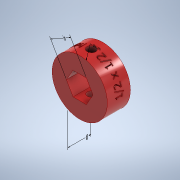
# Autodesk Inventor part: 1_2x1_2x1-1_2HexBearing
Saved by Autodesk Inventor 2022.2 (Build 262287000, 287)
## iProperties
Created: 2020-11-08
Part Number: 1_2x1_2x1-1_2HexBearing
Material: PC/ABS Plastic
Document SubType Name: Modeling
Designer: robst
Density: 0.357273 g/cm^3
Appearance: Red
Author: robst
Autodesk Inventor part; units mm, degrees
ref_plane "YZ Plane" through (0, 0, 0) normal (1, 0, 0) x (0, 1, 0)
ref_plane "XZ Plane" through (0, 0, 0) normal (0, 1, 0) x (-1, 0, 0)
ref_plane "XY Plane" through (0, 0, 0) normal (0, 0, 1) x (1, 0, 0)
sketch "Sketch1" plane through (0, 0, 0) normal (0, 0, 1) x (1, 0, 0)
  line L0 (3.6662, 6.35) -> (7.3323, 0)
  line L1 (7.3323, 0) -> (3.6662, -6.35)
  line L2 (3.6662, -6.35) -> (-3.6662, -6.35)
  line L3 (-3.6662, -6.35) -> (-7.3323, 0)
  line L4 (-7.3323, 0) -> (-3.6662, 6.35)
  line L5 (-3.6662, 6.35) -> (3.6662, 6.35)
  circle A0 centre (0, 0) radius 15.2146
  circle A1 centre (0, 0) radius 7.3323 construction
  dimension "d0" = 12.7
  dimension "d2" = 30.4292
  dimension "d3" = 7.8822
  constraints: 12 end point, 3 coincident, 1 centre point, 1 horizontal, 1 horizontal alignment, 15 other
  measures "d0" distance between parallel lines of L2 L5
  measures "d2" diameter of A0
extrude "Extrusion1" add sketch "Sketch1" against normal blind 12.7
ref_plane "Work Plane1" through (0, 15.2146, 0) normal (0, 1, 0) x (-1, 0, 0)
sketch "Sketch2" plane through (0, 15.2146, 0) normal (0, 1, 0) x (-1, 0, 0)
  line L0 (0, -6.35) -> (-25.4, -6.35) construction
  line L1 (15.2146, 0) -> (-15.2146, 0) construction
  line L2 (-22.9639, -8.255) -> (-24.8226, -8.255)
  line L3 (-24.8226, -8.255) -> (-24.8226, -7.866)
  line L4 (-24.8226, -7.866) -> (-24.131, -7.866)
  line L5 (-24.131, -7.866) -> (-24.131, -5.3126)
  line L6 (-24.131, -5.3126) -> (-24.8226, -5.3126)
  line L7 (-24.8226, -5.3126) -> (-24.8226, -4.9637)
  spline S0 degree 2 poles (-24.8226, -4.9637) (-24.4305, -4.9637) (-24.06, -4.7414) (-24.0353, -4.4326) knots 0 0 0 1 2 2 2
  line L8 (-24.0353, -4.4326) -> (-23.6401, -4.4326)
  line L9 (-23.6401, -4.4326) -> (-23.6401, -7.866)
  line L10 (-23.6401, -7.866) -> (-22.9639, -7.866)
  line L11 (-22.9639, -7.866) -> (-22.9639, -8.255)
  line L12 (-20.6792, -4.2752) -> (-22.1705, -9.0825)
  line L13 (-22.1705, -9.0825) -> (-22.6027, -9.0825)
  line L14 (-22.6027, -9.0825) -> (-21.1176, -4.2752)
  line L15 (-21.1176, -4.2752) -> (-20.6792, -4.2752)
  line L16 (-17.9097, -8.255) -> (-20.2593, -8.255)
  line L17 (-20.2593, -8.255) -> (-20.2593, -7.7147)
  spline S1 degree 2 poles (-20.2593, -7.7147) (-20.0061, -7.4769) (-19.5553, -7.0354) (-19.3392, -6.7977) knots 0 0 0 1 2 2 2
  spline S2 degree 2 poles (-19.3392, -6.7977) (-18.9039, -6.3191) (-18.5858, -5.7448) (-18.5858, -5.4392) knots 0 0 0 1 2 2 2
  spline S3 degree 2 poles (-18.5858, -5.4392) (-18.5858, -5.2786) (-18.6846, -5.0378) (-18.7742, -4.9606) knots 0 0 0 1 2 2 2
  spline S4 degree 2 poles (-18.7742, -4.9606) (-18.8637, -4.8834) (-19.0984, -4.8062) (-19.2404, -4.8062) knots 0 0 0 1 2 2 2
  spline S5 degree 2 poles (-19.2404, -4.8062) (-19.3762, -4.8062) (-19.6541, -4.8742) (-19.7807, -4.9267) knots 0 0 0 1 2 2 2
  spline S6 degree 2 poles (-19.7807, -4.9267) (-19.8888, -4.9699) (-20.0895, -5.0934) (-20.1512, -5.1366) knots 0 0 0 1 2 2 2
  line L18 (-20.1512, -5.1366) -> (-20.179, -5.1366)
  line L19 (-20.179, -5.1366) -> (-20.179, -4.5932)
  spline S7 degree 2 poles (-20.179, -4.5932) (-20.0215, -4.516) (-19.4565, -4.3647) (-19.2033, -4.3647) knots 0 0 0 1 2 2 2
  spline S8 degree 2 poles (-19.2033, -4.3647) (-18.6692, -4.3647) (-18.0671, -4.9297) (-18.0671, -5.4114) knots 0 0 0 1 2 2 2
  spline S9 degree 2 poles (-18.0671, -5.4114) (-18.0671, -5.6368) (-18.1721, -6.0135) (-18.2647, -6.174) knots 0 0 0 1 2 2 2
  spline S10 degree 2 poles (-18.2647, -6.174) (-18.3574, -6.3407) (-18.626, -6.668) (-18.7742, -6.8255) knots 0 0 0 1 2 2 2
  spline S11 degree 2 poles (-18.7742, -6.8255) (-19.015, -7.0879) (-19.6047, -7.6498) (-19.7807, -7.8135) knots 0 0 0 1 2 2 2
  line L20 (-19.7807, -7.8135) -> (-17.9097, -7.8135)
  line L21 (-17.9097, -7.8135) -> (-17.9097, -8.255)
  line L22 (-13.4729, -8.255) -> (-14.0626, -8.255)
  line L23 (-14.0626, -8.255) -> (-14.7573, -7.1805)
  line L24 (-14.7573, -7.1805) -> (-15.4705, -8.255)
  line L25 (-15.4705, -8.255) -> (-16.017, -8.255)
  line L26 (-16.017, -8.255) -> (-15.0259, -6.8378)
  line L27 (-15.0259, -6.8378) -> (-16.0078, -5.396)
  line L28 (-16.0078, -5.396) -> (-15.418, -5.396)
  line L29 (-15.418, -5.396) -> (-14.7264, -6.4612)
  line L30 (-14.7264, -6.4612) -> (-14.0194, -5.396)
  line L31 (-14.0194, -5.396) -> (-13.4729, -5.396)
  line L32 (-13.4729, -5.396) -> (-14.4578, -6.807)
  line L33 (-14.4578, -6.807) -> (-13.4729, -8.255)
  line L34 (-9.3758, -8.255) -> (-11.2345, -8.255)
  line L35 (-11.2345, -8.255) -> (-11.2345, -7.866)
  line L36 (-11.2345, -7.866) -> (-10.5429, -7.866)
  line L37 (-10.5429, -7.866) -> (-10.5429, -5.3126)
  line L38 (-10.5429, -5.3126) -> (-11.2345, -5.3126)
  line L39 (-11.2345, -5.3126) -> (-11.2345, -4.9637)
  spline S12 degree 2 poles (-11.2345, -4.9637) (-10.8423, -4.9637) (-10.4718, -4.7414) (-10.4471, -4.4326) knots 0 0 0 1 2 2 2
  line L40 (-10.4471, -4.4326) -> (-10.0519, -4.4326)
  line L41 (-10.0519, -4.4326) -> (-10.0519, -7.866)
  line L42 (-10.0519, -7.866) -> (-9.3758, -7.866)
  line L43 (-9.3758, -7.866) -> (-9.3758, -8.255)
  line L44 (-7.091, -4.2752) -> (-8.5823, -9.0825)
  line L45 (-8.5823, -9.0825) -> (-9.0145, -9.0825)
  line L46 (-9.0145, -9.0825) -> (-7.5294, -4.2752)
  line L47 (-7.5294, -4.2752) -> (-7.091, -4.2752)
  line L48 (-4.3215, -8.255) -> (-6.6711, -8.255)
  line L49 (-6.6711, -8.255) -> (-6.6711, -7.7147)
  spline S13 degree 2 poles (-6.6711, -7.7147) (-6.4179, -7.4769) (-5.9671, -7.0354) (-5.751, -6.7977) knots 0 0 0 1 2 2 2
  spline S14 degree 2 poles (-5.751, -6.7977) (-5.3157, -6.3191) (-4.9977, -5.7448) (-4.9977, -5.4392) knots 0 0 0 1 2 2 2
  spline S15 degree 2 poles (-4.9977, -5.4392) (-4.9977, -5.2786) (-5.0965, -5.0378) (-5.186, -4.9606) knots 0 0 0 1 2 2 2
  spline S16 degree 2 poles (-5.186, -4.9606) (-5.2755, -4.8834) (-5.5102, -4.8062) (-5.6522, -4.8062) knots 0 0 0 1 2 2 2
  spline S17 degree 2 poles (-5.6522, -4.8062) (-5.7881, -4.8062) (-6.0659, -4.8742) (-6.1925, -4.9267) knots 0 0 0 1 2 2 2
  spline S18 degree 2 poles (-6.1925, -4.9267) (-6.3006, -4.9699) (-6.5013, -5.0934) (-6.563, -5.1366) knots 0 0 0 1 2 2 2
  line L50 (-6.563, -5.1366) -> (-6.5908, -5.1366)
  line L51 (-6.5908, -5.1366) -> (-6.5908, -4.5932)
  spline S19 degree 2 poles (-6.5908, -4.5932) (-6.4334, -4.516) (-5.8683, -4.3647) (-5.6152, -4.3647) knots 0 0 0 1 2 2 2
  spline S20 degree 2 poles (-5.6152, -4.3647) (-5.081, -4.3647) (-4.479, -4.9297) (-4.479, -5.4114) knots 0 0 0 1 2 2 2
  spline S21 degree 2 poles (-4.479, -5.4114) (-4.479, -5.6368) (-4.5839, -6.0135) (-4.6766, -6.174) knots 0 0 0 1 2 2 2
  spline S22 degree 2 poles (-4.6766, -6.174) (-4.7692, -6.3407) (-5.0378, -6.668) (-5.186, -6.8255) knots 0 0 0 1 2 2 2
  spline S23 degree 2 poles (-5.186, -6.8255) (-5.4268, -7.0879) (-6.0165, -7.6498) (-6.1925, -7.8135) knots 0 0 0 1 2 2 2
  line L52 (-6.1925, -7.8135) -> (-4.3215, -7.8135)
  line L53 (-4.3215, -7.8135) -> (-4.3215, -8.255)
  line L54 (6.6855, -8.255) -> (6.2039, -8.255)
  line L55 (6.2039, -8.255) -> (6.2039, -6.6248)
  spline S24 degree 2 poles (6.2039, -6.6248) (6.2039, -6.4272) (6.1668, -6.0876) (6.1112, -5.9857) knots 0 0 0 1 2 2 2
  spline S25 degree 2 poles (6.1112, -5.9857) (6.0526, -5.8776) (5.8426, -5.7726) (5.6635, -5.7726) knots 0 0 0 1 2 2 2
  spline S26 degree 2 poles (5.6635, -5.7726) (5.4845, -5.7726) (5.1047, -5.9641) (4.9225, -6.1184) knots 0 0 0 1 2 2 2
  line L56 (4.9225, -6.1184) -> (4.9225, -8.255)
  line L57 (4.9225, -8.255) -> (4.4409, -8.255)
  line L58 (4.4409, -8.255) -> (4.4409, -4.2752)
  line L59 (4.4409, -4.2752) -> (4.9225, -4.2752)
  line L60 (4.9225, -4.2752) -> (4.9225, -5.714)
  spline S27 degree 2 poles (4.9225, -5.714) (5.1387, -5.5195) (5.5555, -5.3157) (5.7901, -5.3157) knots 0 0 0 1 2 2 2
  spline S28 degree 2 poles (5.7901, -5.3157) (6.21, -5.3157) (6.6855, -5.8714) (6.6855, -6.3994) knots 0 0 0 1 2 2 2
  line L61 (6.6855, -6.3994) -> (6.6855, -8.255)
  spline S29 degree 2 poles (8.6029, -8.3198) (7.9174, -8.3198) (7.1641, -7.551) (7.1641, -6.8409) knots 0 0 0 1 2 2 2
  spline S30 degree 2 poles (7.1641, -6.8409) (7.1641, -6.1431) (7.8958, -5.3157) (8.4855, -5.3157) knots 0 0 0 1 2 2 2
  spline S31 degree 2 poles (8.4855, -5.3157) (8.7511, -5.3157) (9.1617, -5.4701) (9.313, -5.6337) knots 0 0 0 1 2 2 2
  spline S32 degree 2 poles (9.313, -5.6337) (9.4674, -5.7973) (9.631, -6.2697) (9.631, -6.6124) knots 0 0 0 1 2 2 2
  line L62 (9.631, -6.6124) -> (9.631, -6.8749)
  line L63 (9.631, -6.8749) -> (7.6519, -6.8749)
  spline S33 degree 2 poles (7.6519, -6.8749) (7.6519, -7.372) (8.1521, -7.8999) (8.5967, -7.8999) knots 0 0 0 1 2 2 2
  spline S34 degree 2 poles (8.5967, -7.8999) (8.7541, -7.8999) (9.0598, -7.8289) (9.1833, -7.7733) knots 0 0 0 1 2 2 2
  spline S35 degree 2 poles (9.1833, -7.7733) (9.313, -7.7116) (9.4921, -7.6035) (9.5507, -7.5541) knots 0 0 0 1 2 2 2
  line L64 (9.5507, -7.5541) -> (9.5785, -7.5541)
  line L65 (9.5785, -7.5541) -> (9.5785, -8.079)
  spline S36 degree 2 poles (9.5785, -8.079) (9.4952, -8.113) (9.242, -8.2118) (9.1432, -8.2396) knots 0 0 0 1 2 2 2
  spline S37 degree 2 poles (9.1432, -8.2396) (9.0042, -8.2797) (8.7758, -8.3198) (8.6029, -8.3198) knots 0 0 0 1 2 2 2
  spline S38 degree 2 poles (9.1617, -6.5075) (9.1555, -6.3129) (9.0753, -6.0289) (8.9981, -5.9332) knots 0 0 0 1 2 2 2
  spline S39 degree 2 poles (8.9981, -5.9332) (8.9147, -5.8251) (8.6523, -5.7109) (8.4577, -5.7109) knots 0 0 0 1 2 2 2
  spline S40 degree 2 poles (8.4577, -5.7109) (8.2663, -5.7109) (7.9977, -5.8251) (7.8866, -5.9363) knots 0 0 0 1 2 2 2
  spline S41 degree 2 poles (7.8866, -5.9363) (7.7785, -6.0505) (7.6673, -6.3253) (7.6519, -6.5075) knots 0 0 0 1 2 2 2
  line L66 (7.6519, -6.5075) -> (9.1617, -6.5075)
  line L67 (12.3388, -8.255) -> (11.749, -8.255)
  line L68 (11.749, -8.255) -> (11.0544, -7.1805)
  line L69 (11.0544, -7.1805) -> (10.3411, -8.255)
  line L70 (10.3411, -8.255) -> (9.7946, -8.255)
  line L71 (9.7946, -8.255) -> (10.7857, -6.8378)
  line L72 (10.7857, -6.8378) -> (9.8039, -5.396)
  line L73 (9.8039, -5.396) -> (10.3936, -5.396)
  line L74 (10.3936, -5.396) -> (11.0852, -6.4612)
  line L75 (11.0852, -6.4612) -> (11.7923, -5.396)
  line L76 (11.7923, -5.396) -> (12.3388, -5.396)
  line L77 (12.3388, -5.396) -> (11.3538, -6.807)
  line L78 (11.3538, -6.807) -> (12.3388, -8.255)
  spline S42 degree 2 poles (16.7447, -6.7792) (16.7447, -7.48) (16.0654, -8.3353) (15.5529, -8.3353) knots 0 0 0 1 2 2 2
  spline S43 degree 2 poles (15.5529, -8.3353) (15.3213, -8.3353) (14.9909, -8.221) (14.8304, -8.1222) knots 0 0 0 1 2 2 2
  line L79 (14.8304, -8.1222) -> (14.7995, -8.255)
  line L80 (14.7995, -8.255) -> (14.3487, -8.255)
  line L81 (14.3487, -8.255) -> (14.3487, -4.2752)
  line L82 (14.3487, -4.2752) -> (14.8304, -4.2752)
  line L83 (14.8304, -4.2752) -> (14.8304, -5.6954)
  spline S44 degree 2 poles (14.8304, -5.6954) (15.0126, -5.5318) (15.4355, -5.3157) (15.7042, -5.3157) knots 0 0 0 1 2 2 2
  spline S45 degree 2 poles (15.7042, -5.3157) (16.1889, -5.3157) (16.7447, -6.0906) (16.7447, -6.7792) knots 0 0 0 1 2 2 2
  spline S46 degree 2 poles (16.2476, -6.8162) (16.2476, -6.3037) (15.9357, -5.7726) (15.5899, -5.7726) knots 0 0 0 1 2 2 2
  spline S47 degree 2 poles (15.5899, -5.7726) (15.3954, -5.7726) (14.994, -5.9579) (14.8304, -6.0999) knots 0 0 0 1 2 2 2
  line L84 (14.8304, -6.0999) -> (14.8304, -7.7394)
  spline S48 degree 2 poles (14.8304, -7.7394) (15.0126, -7.8289) (15.2935, -7.903) (15.4602, -7.903) knots 0 0 0 1 2 2 2
  spline S49 degree 2 poles (15.4602, -7.903) (15.8277, -7.903) (16.2476, -7.3812) (16.2476, -6.8162) knots 0 0 0 1 2 2 2
  line L85 (19.4678, -8.255) -> (18.9862, -8.255)
  line L86 (18.9862, -8.255) -> (18.9862, -7.9401)
  spline S50 degree 2 poles (18.9862, -7.9401) (18.7639, -8.1346) (18.3656, -8.3353) (18.1186, -8.3353) knots 0 0 0 1 2 2 2
  spline S51 degree 2 poles (18.1186, -8.3353) (17.9333, -8.3353) (17.603, -8.2118) (17.4826, -8.079) knots 0 0 0 1 2 2 2
  spline S52 degree 2 poles (17.4826, -8.079) (17.3591, -7.9462) (17.2232, -7.5418) (17.2232, -7.2516) knots 0 0 0 1 2 2 2
  line L87 (17.2232, -7.2516) -> (17.2232, -5.396)
  line L88 (17.2232, -5.396) -> (17.7049, -5.396)
  line L89 (17.7049, -5.396) -> (17.7049, -7.0262)
  spline S53 degree 2 poles (17.7049, -7.0262) (17.7049, -7.2546) (17.7388, -7.5541) (17.7975, -7.6653) knots 0 0 0 1 2 2 2
  spline S54 degree 2 poles (17.7975, -7.6653) (17.8562, -7.7764) (18.0568, -7.8783) (18.2452, -7.8783) knots 0 0 0 1 2 2 2
  spline S55 degree 2 poles (18.2452, -7.8783) (18.4212, -7.8783) (18.8195, -7.6776) (18.9862, -7.5325) knots 0 0 0 1 2 2 2
  line L90 (18.9862, -7.5325) -> (18.9862, -5.396)
  line L91 (18.9862, -5.396) -> (19.4678, -5.396)
  line L92 (19.4678, -5.396) -> (19.4678, -8.255)
  spline S56 degree 2 poles (20.9375, -8.3229) (20.6504, -8.3229) (20.1533, -8.1685) (19.9896, -8.0821) knots 0 0 0 1 2 2 2
  line L93 (19.9896, -8.0821) -> (19.9896, -7.5418)
  line L94 (19.9896, -7.5418) -> (20.0143, -7.5418)
  spline S57 degree 2 poles (20.0143, -7.5418) (20.0761, -7.5912) (20.2428, -7.7085) (20.3818, -7.7733) knots 0 0 0 1 2 2 2
  spline S58 degree 2 poles (20.3818, -7.7733) (20.5022, -7.832) (20.7986, -7.9185) (20.956, -7.9185) knots 0 0 0 1 2 2 2
  spline S59 degree 2 poles (20.956, -7.9185) (21.0703, -7.9185) (21.3327, -7.866) (21.3945, -7.8227) knots 0 0 0 1 2 2 2
  spline S60 degree 2 poles (21.3945, -7.8227) (21.484, -7.7641) (21.5643, -7.6313) (21.5643, -7.4955) knots 0 0 0 1 2 2 2
  spline S61 degree 2 poles (21.5643, -7.4955) (21.5643, -7.3257) (21.379, -7.1497) (21.1413, -7.091) knots 0 0 0 1 2 2 2
  spline S62 degree 2 poles (21.1413, -7.091) (21.0487, -7.0694) (20.7523, -7.0076) (20.6257, -6.9737) knots 0 0 0 1 2 2 2
  spline S63 degree 2 poles (20.6257, -6.9737) (20.2984, -6.878) (20.002, -6.4828) (20.002, -6.2018) knots 0 0 0 1 2 2 2
  spline S64 degree 2 poles (20.002, -6.2018) (20.002, -5.8128) (20.5855, -5.328) (21.0672, -5.328) knots 0 0 0 1 2 2 2
  spline S65 degree 2 poles (21.0672, -5.328) (21.3049, -5.328) (21.7866, -5.4454) (21.9502, -5.5349) knots 0 0 0 1 2 2 2
  line L95 (21.9502, -5.5349) -> (21.9502, -6.0505)
  line L96 (21.9502, -6.0505) -> (21.9255, -6.0505)
  spline S66 degree 2 poles (21.9255, -6.0505) (21.7403, -5.9023) (21.2895, -5.7325) (21.0579, -5.7325) knots 0 0 0 1 2 2 2
  spline S67 degree 2 poles (21.0579, -5.7325) (20.8202, -5.7325) (20.4929, -5.9332) (20.4929, -6.1339) knots 0 0 0 1 2 2 2
  spline S68 degree 2 poles (20.4929, -6.1339) (20.4929, -6.316) (20.6874, -6.492) (20.9035, -6.5476) knots 0 0 0 1 2 2 2
  spline S69 degree 2 poles (20.9035, -6.5476) (21.0085, -6.5754) (21.274, -6.631) (21.4192, -6.6649) knots 0 0 0 1 2 2 2
  spline S70 degree 2 poles (21.4192, -6.6649) (21.7341, -6.7452) (22.0552, -7.1126) (22.0552, -7.4306) knots 0 0 0 1 2 2 2
  spline S71 degree 2 poles (22.0552, -7.4306) (22.0552, -7.6159) (21.9101, -7.9432) (21.768, -8.0636) knots 0 0 0 1 2 2 2
  spline S72 degree 2 poles (21.768, -8.0636) (21.6168, -8.1902) (21.2308, -8.3229) (20.9375, -8.3229) knots 0 0 0 1 2 2 2
  line L97 (24.7475, -8.255) -> (24.2659, -8.255)
  line L98 (24.2659, -8.255) -> (24.2659, -6.6248)
  spline S73 degree 2 poles (24.2659, -6.6248) (24.2659, -6.4272) (24.2288, -6.0876) (24.1732, -5.9857) knots 0 0 0 1 2 2 2
  spline S74 degree 2 poles (24.1732, -5.9857) (24.1146, -5.8776) (23.9046, -5.7726) (23.7255, -5.7726) knots 0 0 0 1 2 2 2
  spline S75 degree 2 poles (23.7255, -5.7726) (23.5465, -5.7726) (23.1667, -5.9641) (22.9845, -6.1184) knots 0 0 0 1 2 2 2
  line L99 (22.9845, -6.1184) -> (22.9845, -8.255)
  line L100 (22.9845, -8.255) -> (22.5029, -8.255)
  line L101 (22.5029, -8.255) -> (22.5029, -4.2752)
  line L102 (22.5029, -4.2752) -> (22.9845, -4.2752)
  line L103 (22.9845, -4.2752) -> (22.9845, -5.714)
  spline S76 degree 2 poles (22.9845, -5.714) (23.2007, -5.5195) (23.6175, -5.3157) (23.8521, -5.3157) knots 0 0 0 1 2 2 2
  spline S77 degree 2 poles (23.8521, -5.3157) (24.272, -5.3157) (24.7475, -5.8714) (24.7475, -6.3994) knots 0 0 0 1 2 2 2
  line L104 (24.7475, -6.3994) -> (24.7475, -8.255)
  line L105 (25.9146, -8.255) -> (25.4329, -8.255)
  line L106 (25.4329, -8.255) -> (25.4329, -5.396)
  line L107 (25.4329, -5.396) -> (25.9146, -5.396)
  line L108 (25.9146, -5.396) -> (25.9146, -8.255)
  line L109 (25.9486, -4.9205) -> (25.4021, -4.9205)
  line L110 (25.4021, -4.9205) -> (25.4021, -4.4203)
  line L111 (25.4021, -4.4203) -> (25.9486, -4.4203)
  line L112 (25.9486, -4.4203) -> (25.9486, -4.9205)
  line L113 (28.8663, -8.255) -> (28.3846, -8.255)
  line L114 (28.3846, -8.255) -> (28.3846, -6.6248)
  spline S78 degree 2 poles (28.3846, -6.6248) (28.3846, -6.4272) (28.3476, -6.0876) (28.292, -5.9857) knots 0 0 0 1 2 2 2
  spline S79 degree 2 poles (28.292, -5.9857) (28.2333, -5.8776) (28.0234, -5.7726) (27.8443, -5.7726) knots 0 0 0 1 2 2 2
  spline S80 degree 2 poles (27.8443, -5.7726) (27.6652, -5.7726) (27.2854, -5.9641) (27.1033, -6.1184) knots 0 0 0 1 2 2 2
  line L115 (27.1033, -6.1184) -> (27.1033, -8.255)
  line L116 (27.1033, -8.255) -> (26.6216, -8.255)
  line L117 (26.6216, -8.255) -> (26.6216, -5.396)
  line L118 (26.6216, -5.396) -> (27.1033, -5.396)
  line L119 (27.1033, -5.396) -> (27.1033, -5.714)
  spline S81 degree 2 poles (27.1033, -5.714) (27.3194, -5.5195) (27.7362, -5.3157) (27.9709, -5.3157) knots 0 0 0 1 2 2 2
  spline S82 degree 2 poles (27.9709, -5.3157) (28.3908, -5.3157) (28.8663, -5.8714) (28.8663, -6.3994) knots 0 0 0 1 2 2 2
  line L120 (28.8663, -6.3994) -> (28.8663, -8.255)
  spline S83 degree 2 poles (29.6443, -8.712) (29.6937, -8.7336) (29.8821, -8.8015) (30.0025, -8.8293) knots 0 0 0 1 2 2 2
  spline S84 degree 2 poles (30.0025, -8.8293) (30.1352, -8.8632) (30.3606, -8.9034) (30.4934, -8.9034) knots 0 0 0 1 2 2 2
  spline S85 degree 2 poles (30.4934, -8.9034) (30.7157, -8.9034) (31.0244, -8.7861) (31.1109, -8.6811) knots 0 0 0 1 2 2 2
  spline S86 degree 2 poles (31.1109, -8.6811) (31.1942, -8.5761) (31.2591, -8.3013) (31.2591, -8.1253) knots 0 0 0 1 2 2 2
  line L121 (31.2591, -8.1253) -> (31.2591, -7.8752)
  spline S87 degree 2 poles (31.2591, -7.8752) (31.0646, -8.045) (30.691, -8.2056) (30.41, -8.2056) knots 0 0 0 1 2 2 2
  spline S88 degree 2 poles (30.41, -8.2056) (29.9222, -8.2056) (29.3448, -7.48) (29.3448, -6.7977) knots 0 0 0 1 2 2 2
  spline S89 degree 2 poles (29.3448, -6.7977) (29.3448, -6.4426) (29.5455, -5.893) (29.7122, -5.6985) knots 0 0 0 1 2 2 2
  spline S90 degree 2 poles (29.7122, -5.6985) (29.8728, -5.5164) (30.3143, -5.3157) (30.549, -5.3157) knots 0 0 0 1 2 2 2
  spline S91 degree 2 poles (30.549, -5.3157) (30.7713, -5.3157) (31.0954, -5.4207) (31.2591, -5.5164) knots 0 0 0 1 2 2 2
  line L122 (31.2591, -5.5164) -> (31.2869, -5.396)
  line L123 (31.2869, -5.396) -> (31.7407, -5.396)
  line L124 (31.7407, -5.396) -> (31.7407, -7.9277)
  spline S92 degree 2 poles (31.7407, -7.9277) (31.7407, -8.6564) (31.1078, -9.3356) (30.4563, -9.3356) knots 0 0 0 1 2 2 2
  spline S93 degree 2 poles (30.4563, -9.3356) (30.2464, -9.3356) (29.808, -9.2677) (29.6196, -9.2121) knots 0 0 0 1 2 2 2
  line L125 (29.6196, -9.2121) -> (29.6196, -8.712)
  line L126 (29.6196, -8.712) -> (29.6443, -8.712)
  line L127 (31.2591, -7.48) -> (31.2591, -5.9085)
  spline S94 degree 2 poles (31.2591, -5.9085) (31.08, -5.822) (30.7774, -5.7479) (30.6261, -5.7479) knots 0 0 0 1 2 2 2
  spline S95 degree 2 poles (30.6261, -5.7479) (30.2618, -5.7479) (29.8419, -6.2852) (29.8419, -6.7884) knots 0 0 0 1 2 2 2
  spline S96 degree 2 poles (29.8419, -6.7884) (29.8419, -7.2639) (30.1599, -7.761) (30.5181, -7.761) knots 0 0 0 1 2 2 2
  spline S97 degree 2 poles (30.5181, -7.761) (30.7064, -7.761) (31.1016, -7.6128) (31.2591, -7.48) knots 0 0 0 1 2 2 2
  spline S98 degree 2 poles (36.4708, -6.7483) (36.4708, -7.4646) (35.7885, -8.3106) (35.2667, -8.3106) knots 0 0 0 1 2 2 2
  spline S99 degree 2 poles (35.2667, -8.3106) (35.0536, -8.3106) (34.7264, -8.2118) (34.5566, -8.1099) knots 0 0 0 1 2 2 2
  line L128 (34.5566, -8.1099) -> (34.5566, -9.3078)
  line L129 (34.5566, -9.3078) -> (34.0749, -9.3078)
  line L130 (34.0749, -9.3078) -> (34.0749, -5.396)
  line L131 (34.0749, -5.396) -> (34.5566, -5.396)
  line L132 (34.5566, -5.396) -> (34.5566, -5.6954)
  spline S100 degree 2 poles (34.5566, -5.6954) (34.7356, -5.5318) (35.1741, -5.3157) (35.4303, -5.3157) knots 0 0 0 1 2 2 2
  spline S101 degree 2 poles (35.4303, -5.3157) (35.9212, -5.3157) (36.4708, -6.0937) (36.4708, -6.7483) knots 0 0 0 1 2 2 2
  spline S102 degree 2 poles (35.9737, -6.8039) (35.9737, -6.3129) (35.6619, -5.7726) (35.313, -5.7726) knots 0 0 0 1 2 2 2
  spline S103 degree 2 poles (35.313, -5.7726) (35.1092, -5.7726) (34.7264, -5.9548) (34.5566, -6.0968) knots 0 0 0 1 2 2 2
  line L133 (34.5566, -6.0968) -> (34.5566, -7.7209)
  spline S104 degree 2 poles (34.5566, -7.7209) (34.7449, -7.8104) (35.0135, -7.8783) (35.1864, -7.8783) knots 0 0 0 1 2 2 2
  spline S105 degree 2 poles (35.1864, -7.8783) (35.56, -7.8783) (35.9737, -7.3287) (35.9737, -6.8039) knots 0 0 0 1 2 2 2
  line L134 (39.2156, -5.396) -> (38.1381, -8.255)
  line L135 (38.1381, -8.255) -> (37.7058, -8.255)
  line L136 (37.7058, -8.255) -> (36.6375, -5.396)
  line L137 (36.6375, -5.396) -> (37.1593, -5.396)
  line L138 (37.1593, -5.396) -> (37.9405, -7.5974)
  line L139 (37.9405, -7.5974) -> (38.7154, -5.396)
  line L140 (38.7154, -5.396) -> (39.2156, -5.396)
  spline S106 degree 2 poles (41.8802, -6.35) (41.8802, -7.3751) (41.2843, -8.3353) (40.6637, -8.3353) knots 0 0 0 1 2 2 2
  spline S107 degree 2 poles (40.6637, -8.3353) (40.0338, -8.3353) (39.4441, -7.3565) (39.4441, -6.3531) knots 0 0 0 1 2 2 2
  spline S108 degree 2 poles (39.4441, -6.3531) (39.4441, -5.3219) (40.04, -4.3678) (40.6637, -4.3678) knots 0 0 0 1 2 2 2
  spline S109 degree 2 poles (40.6637, -4.3678) (41.2904, -4.3678) (41.8802, -5.3558) (41.8802, -6.35) knots 0 0 0 1 2 2 2
  spline S110 degree 2 poles (41.2256, -7.5109) (41.2997, -7.3226) (41.3615, -6.7421) (41.3615, -6.35) knots 0 0 0 1 2 2 2
  spline S111 degree 2 poles (41.3615, -6.35) (41.3615, -5.9579) (41.2997, -5.3805) (41.2225, -5.186) knots 0 0 0 1 2 2 2
  spline S112 degree 2 poles (41.2225, -5.186) (41.1453, -4.9915) (40.8767, -4.7908) (40.6637, -4.7908) knots 0 0 0 1 2 2 2
  spline S113 degree 2 poles (40.6637, -4.7908) (40.4506, -4.7908) (40.1758, -4.9915) (40.0956, -5.1922) knots 0 0 0 1 2 2 2
  spline S114 degree 2 poles (40.0956, -5.1922) (40.0184, -5.3867) (39.9628, -5.9795) (39.9628, -6.3531) knots 0 0 0 1 2 2 2
  spline S115 degree 2 poles (39.9628, -6.3531) (39.9628, -6.7545) (40.0122, -7.2917) (40.0925, -7.5016) knots 0 0 0 1 2 2 2
  spline S116 degree 2 poles (40.0925, -7.5016) (40.1666, -7.6992) (40.4414, -7.9123) (40.6637, -7.9123) knots 0 0 0 1 2 2 2
  spline S117 degree 2 poles (40.6637, -7.9123) (40.8736, -7.9123) (41.1484, -7.7116) (41.2256, -7.5109) knots 0 0 0 1 2 2 2
  spline S118 degree 2 poles (43.3961, -4.8062) (43.2572, -4.8062) (42.9824, -4.8742) (42.8496, -4.9267) knots 0 0 0 1 2 2 2
  spline S119 degree 2 poles (42.8496, -4.9267) (42.7261, -4.9791) (42.544, -5.0903) (42.473, -5.1397) knots 0 0 0 1 2 2 2
  line L141 (42.473, -5.1397) -> (42.4421, -5.1397)
  line L142 (42.4421, -5.1397) -> (42.4421, -4.5994)
  spline S120 degree 2 poles (42.4421, -4.5994) (42.6088, -4.5098) (43.18, -4.3647) (43.4363, -4.3647) knots 0 0 0 1 2 2 2
  spline S121 degree 2 poles (43.4363, -4.3647) (43.6956, -4.3647) (44.0816, -4.4697) (44.239, -4.5809) knots 0 0 0 1 2 2 2
  spline S122 degree 2 poles (44.239, -4.5809) (44.4057, -4.7013) (44.5786, -5.0502) (44.5786, -5.2848) knots 0 0 0 1 2 2 2
  spline S123 degree 2 poles (44.5786, -5.2848) (44.5786, -5.5997) (44.1649, -6.0752) (43.8747, -6.137) knots 0 0 0 1 2 2 2
  line L143 (43.8747, -6.137) -> (43.8747, -6.174)
  spline S124 degree 2 poles (43.8747, -6.174) (43.9951, -6.1987) (44.2699, -6.3099) (44.3872, -6.421) knots 0 0 0 1 2 2 2
  spline S125 degree 2 poles (44.3872, -6.421) (44.5045, -6.5291) (44.6527, -6.8749) (44.6527, -7.125) knots 0 0 0 1 2 2 2
  spline S126 degree 2 poles (44.6527, -7.125) (44.6527, -7.3812) (44.4768, -7.8166) (44.3162, -7.9833) knots 0 0 0 1 2 2 2
  spline S127 degree 2 poles (44.3162, -7.9833) (44.1495, -8.1562) (43.6771, -8.3353) (43.3776, -8.3353) knots 0 0 0 1 2 2 2
  spline S128 degree 2 poles (43.3776, -8.3353) (43.0905, -8.3353) (42.5285, -8.1963) (42.3371, -8.1006) knots 0 0 0 1 2 2 2
  line L144 (42.3371, -8.1006) -> (42.3371, -7.5603)
  line L145 (42.3371, -7.5603) -> (42.3742, -7.5603)
  spline S129 degree 2 poles (42.3742, -7.5603) (42.5347, -7.6776) (43.0781, -7.8938) (43.3467, -7.8938) knots 0 0 0 1 2 2 2
  spline S130 degree 2 poles (43.3467, -7.8938) (43.5042, -7.8938) (43.8191, -7.795) (43.9241, -7.6807) knots 0 0 0 1 2 2 2
  spline S131 degree 2 poles (43.9241, -7.6807) (44.026, -7.5665) (44.134, -7.2948) (44.134, -7.0879) knots 0 0 0 1 2 2 2
  spline S132 degree 2 poles (44.134, -7.0879) (44.134, -6.8811) (44.0136, -6.6124) (43.9056, -6.5353) knots 0 0 0 1 2 2 2
  spline S133 degree 2 poles (43.9056, -6.5353) (43.7975, -6.4581) (43.5042, -6.3994) (43.3313, -6.3994) knots 0 0 0 1 2 2 2
  line L146 (43.3313, -6.3994) -> (43.1152, -6.3994)
  line L147 (43.1152, -6.3994) -> (43.1152, -5.9764)
  line L148 (43.1152, -5.9764) -> (43.285, -5.9764)
  spline S134 degree 2 poles (43.285, -5.9764) (43.6277, -5.9764) (44.0599, -5.6491) (44.0599, -5.3373) knots 0 0 0 1 2 2 2
  spline S135 degree 2 poles (44.0599, -5.3373) (44.0599, -5.1922) (43.9488, -4.9853) (43.8593, -4.9236) knots 0 0 0 1 2 2 2
  spline S136 degree 2 poles (43.8593, -4.9236) (43.7635, -4.8587) (43.5289, -4.8062) (43.3961, -4.8062) knots 0 0 0 1 2 2 2
  point P0 (0, 0)
  dimension "d17" = 25.4
  dimension "d18" = 6.35
  constraints: 2 end point, 2 horizontal
  measures "d17" distance of L0.start L0.end
  measures "d18" distance between parallel lines of L0 L1
emboss "Emboss1" sketch "Sketch2" operation cut depth 2.54 direction (0, -1, 0) wrap yes faces at (15.1653, -1.2243, -8.4667)
sketch "Sketch3" plane through (0, 15.2146, 0) normal (0, 1, 0) x (-1, 0, 0)
  line L0 (3.6662, 0) -> (-3.6662, 0) construction
  line L1 (0, 0) -> (0, -12.7) construction
  line L2 (-3.6662, -12.7) -> (3.6662, -12.7) construction
  line L3 (15.2146, 0) -> (-15.2146, 0) projected
  line L4 (-15.2146, -12.7) -> (15.2146, -12.7) projected
  point P0 (0, 0)
  point P1 (0, -6.35)
  dimension "d28" = 6.35
  dimension "d29" = 6.35
  constraints: 3 midpoint, 2 end point
  measures "d28" distance from line of L3 point (0, -6.35)
  measures "d29" distance from line of L4 point (0, -6.35)
hole "Hole1" at (0, 15.2146, -6.35) direction (0, -1, 0) diameter 4.318 end through all clearance for "Hex Machine Screw" size "#6" standard "Ansi Unified Screw Threads"
sketch "Sketch4" plane through (0, 15.2146, 0) normal (0, 1, 0) x (-1, 0, 0)
  circle A0 centre (0, -6.35) radius 2.159 projected
  circle A1 centre (0, -6.35) radius 2.4257
  point P0 (0, 0)
  point P1 (0, -4.445)
  point P2 (2.0138, -5.8255)
  point P3 (2.0136, -7.3829)
  point P4 (1.4342, -8.2178)
  point P5 (-0.3417, -8.7358)
  point P6 (1.6461, -8.001)
  point P7 (1.1668, -8.4205)
  point P8 (1.1668, -4.7875)
  point P9 (1.6461, -5.207)
  point P10 (1.0457, -8.4928)
  point P11 (0.14, -8.7585)
  point P12 (2.125, -6.2226)
  point P13 (-1.8043, -5.4183)
  point P14 (2.1177, -5.93)
  point P15 (0.209, -4.2011)
  point P16 (2.1177, -5.93)
  point P17 (0, -8.763)
  point P18 (0, -4.4768)
  point P19 (0, -8.7948)
  dimension "d30" = 4.8514
  constraints: 1 centre point, 1 coincident, 7 other
  measures "d30" diameter of A1
extrude "Extrusion2" cut sketch "Sketch4" against normal blind 5.5524 contours A0 | A1
ref_plane "Work Plane2" through (0, -15.2146, 0) normal (0, 1, 0) x (-1, 0, 0)
sketch "Sketch5" plane through (0, -15.2146, 0) normal (0, 1, 0) x (-1, 0, 0)
  circle A0 centre (0, -6.35) radius 2.159 projected
  circle A1 centre (0, -6.35) radius 3.429
  point P0 (0, 0)
  point P1 (0.9744, -4.4234)
  dimension "d33" = 6.858
  constraints: 1 centre point, 1 coincident, 1 other
  measures "d33" diameter of A1
extrude "Extrusion3" cut sketch "Sketch5" along normal blind 1.8542 contours A0 | A1
equation "\"d0\" = hexSize"
equation "\"d2\" = externalDiameter"
equation "\"d4\" = thickness"
equation "\"hexSize\" = 12.7"
equation "\"externalDiameter\" = 30.4292"
equation "\"thickness\" = 12.7"
body "Solid1"
